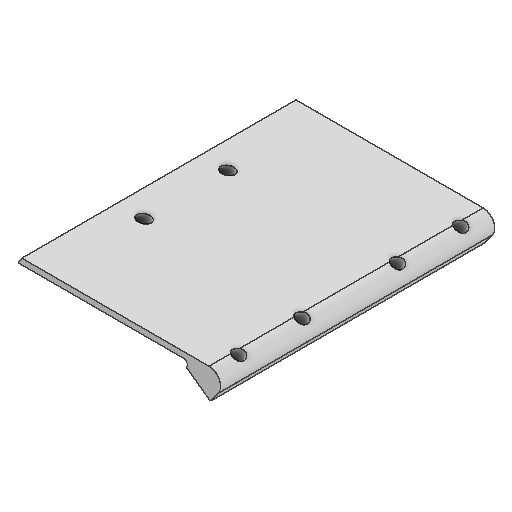
# Autodesk Inventor part: rearSkidPlate
Saved by Autodesk Inventor 2025 (Build 290162000, 162)
## iProperties
Created: 2025-01-06
Part Number: rearSkidPlate
Material: Generic
Document SubType Name: Modeling
Designer: derm
Density: 1 g/cm^3
Appearance: Default
Author: derm
Autodesk Inventor part; units mm, degrees
ref_plane "YZ Plane" through (0, 0, 0) normal (1, 0, 0) x (0, 1, 0)
sketch "Sketch1" plane through (0, 0, 0) normal (0, 1, 0) x (-1, 0, 0)
  line L0 (-60, 117) -> (60, 117)
  line L1 (60, 117) -> (60, -117)
  line L2 (60, -117) -> (-60, -117)
  line L3 (-60, -117) -> (-60, 117)
  line L4 (-60, 117) -> (60, -117) construction
  line L5 (60, 117) -> (-60, -117) construction
  point P0 (0, 0)
  dimension "d0" = 234
  dimension "d1" = 120
  constraints: 12 end point, 2 midpoint, 2 parallel, 1 horizontal, 1 perpendicular
  measures "d0" distance of L2.end L0.start
  measures "d1" distance of L1.end L2.end
extrude "Extrusion1" add sketch "Sketch1" along normal blind 5
sketch "Sketch2" plane through (60, 0, -117) normal (0, 0, -1) x (-1, 0, 0)
  line L0 (220.5261, -138.6359) -> (120, 0) projected
  line L1 (0, 0) -> (120, 0) projected
  line L2 (120, 0) -> (120, 5) projected
  line L3 (0, 5) -> (120, 5) projected
  line L4 (0, 0) -> (0, 5) projected
  line L5 (120, 0) -> (116.3745, 5)
  point P0 (60, 0)
  constraints: 2 end point, 1 point on line
extrude "Extrusion2" cut sketch "Sketch2" against normal through all contours L5 L3 L2
sketch "Sketch3" plane through (60, 0, -117) normal (0, 0, -1) x (-1, 0, 0)
  line L0 (120, 0) -> (116.3745, 5) projected
  line L1 (0, 5) -> (116.3745, 5) projected
  line L2 (0, 0) -> (0, 5) projected
  line L3 (0, 0) -> (120, 0) projected
  line L4 (-29.1464, -9.1279) -> (-26.3491, -7.0996) projected
  line L5 (-44.5674, -20.3098) -> (-40.8398, -25.4506) projected
  line L6 (0, 5) -> (-62.9198, 5)
  line L7 (0, 0) -> (-27.9195, 0)
  line L8 (-79.2318, 0) -> (-79.2318, 5)
  line L9 (-9.681, -25.1528) -> (-22.4191, -7.5856) projected
  line L10 (-22.4191, -7.5856) -> (-27.9195, 0)
  line L11 (-44.5674, -20.3098) -> (-62.9198, 5)
  line L12 (-24.0044, -5.3994) -> (-44.5674, -20.3098)
  line L13 (-8.3183, -25.4) -> (-8.3183, -2.8036) projected
  line L14 (-8.3183, 0) -> (-8.3183, -25.4)
  line L15 (-8.3183, -25.4) -> (-9.0939, -25.9624)
  line L16 (-9.0939, -25.9624) -> (-27.9195, 0)
  point P0 (60, 0)
  point P1 (-26.3491, -7.0996)
  constraints: 18 end point, 2 collinear, 2 horizontal, 2 perpendicular, 2 point on line
extrude "Extrusion3" add sketch "Sketch3" against normal up to surface (234 mm away) contours L7 L10 L12 L4 L11 L6 L2 | L14 L13 L15 L16 L9 L10 L7
fillet "Fillet1" radius 10 1 edges at (122.9198, 5, 0)
sketch "Sketch4" plane through (68.3183, 0, -117) normal (0, 0, -1) x (-1, 0, 0)
  arc A0 (-34.9981, 5) -> (-43.0938, -10.8703) centre (-34.9981, -5) ccw projected
  line L0 (-43.0938, -10.8703) -> (-36.2491, -20.3098) projected
  line L1 (-36.2491, -20.3098) -> (-15.6861, -5.3994) projected
  line L2 (-15.6861, -5.3994) -> (-0.7756, -25.9624) projected
  line L3 (-0.7756, -25.9624) -> (0, -25.4) projected
  line L4 (0, -25.4) -> (0, 0) projected
  line L5 (0, 0) -> (128.3183, 0) projected
  line L6 (128.3183, 0) -> (124.6928, 5) projected
  line L7 (124.6928, 5) -> (-34.9981, 5) projected
  line L8 (0, 0) -> (128.3183, 0) projected
  line L9 (0, 0) -> (-19.6012, 0)
  line L10 (-15.6861, -5.3994) -> (-19.6012, 0)
  point P0 (68.3183, 0)
  constraints: 4 end point, 1 horizontal
extrude "Extrusion4" cut sketch "Sketch4" against normal blind 44.45 contours L10 L9 L4 L3 L2
fillet "Fillet2" radius 3 1 edges at (87.9195, 0, -94.775)
mirror "Mirror1" about plane through (0, 0, 0) normal (0, 0, 1) of "Fillet2", "Extrusion4"
sketch "Sketch5" plane through (0, 0, 0) normal (0, 0, 1) x (1, 0, 0)
  line L0 (84.0044, -5.3994) -> (84.4672, -4.7611) projected
  arc A0 (84.4672, -4.7611) -> (82.0385, 0) centre (82.0385, -3) ccw projected
  line L1 (82.0385, 0) -> (-60, 0) projected
  line L2 (-60, 0) -> (-56.3745, 5) projected
  line L3 (-56.3745, 5) -> (103.3164, 5) projected
  arc A1 (111.4121, -10.8703) -> (103.3164, 5) centre (103.3164, -5) ccw projected
  line L4 (111.4121, -10.8703) -> (104.5674, -20.3098) projected
  line L5 (104.5674, -20.3098) -> (84.0044, -5.3994) projected
  line L6 (-59.5814, -11.3472) -> (-46.3045, -20.9744) projected
  line L7 (-52.9392, -0.4835) -> (-155.6686, -142.158) projected
  line L8 (-48.6719, -37.8674) -> (-54.5421, -45.963) projected
  line L9 (-54.5421, -45.963) -> (-39.8279, -25.6706)
  line L10 (-39.8279, -25.6706) -> (-60.391, -10.7602)
  line L11 (-60.391, -10.7602) -> (-52.5886, 0)
  line L12 (82.0385, 0) -> (-60, 0) projected
  line L13 (-39.8279, -25.6706) -> (-21.2139, 0)
  line L14 (-60, 0) -> (82.0385, 0) projected
  line L15 (-52.5886, 0) -> (-21.2139, 0)
  point P0 (0, 0)
  constraints: 10 end point, 3 point on line, 1 collinear, 1 perpendicular
extrude "Extrusion5" add sketch "Sketch5" along normal mid plane 101.6 contours L13 L10 L6 L7 L11 L1
sketch "Sketch6" plane through (-39.8279, -25.6706, -50.8) normal (-0.5870252, -0.8095687, 0) x (0.8095687, -0.5870252, 0)
  line L0 (0, 0) -> (0, 101.6) projected
  line L1 (-25.4, 101.6) -> (0, 101.6) projected
  line L2 (-25.4, 0) -> (-25.4, 101.6) projected
  line L3 (0, 0) -> (-25.4, 0) projected
  line L4 (88.351, 167.8) -> (113.751, 167.8) projected
  line L5 (88.351, 123.35) -> (88.351, 167.8) projected
  line L6 (88.351, -21.75) -> (88.351, 123.35) projected
  line L7 (88.351, -66.2) -> (88.351, -21.75) projected
  line L8 (113.751, -66.2) -> (88.351, -66.2) projected
  line L9 (113.751, -66.2) -> (113.751, 167.8) projected
  line L10 (113.751, 50.8) -> (-31.4, 50.8) construction
  line L11 (-31.4, -66.2) -> (-31.4, 167.8) projected
  circle A0 centre (-12.7, 86.5239) radius 2.75
  circle A1 centre (101.051, 145.575) radius 2.75
  circle A2 centre (101.051, 91.4911) radius 2.75
  circle A3 centre (-12.7, 15.0761) radius 2.75
  circle A4 centre (101.051, -43.975) radius 2.75
  circle A5 centre (101.051, 10.1089) radius 2.75
  point P0 (17.1741, 50.8)
  dimension "d14" = 5.5
  constraints: 6 centre point, 3 symmetric about line, 2 end point, 2 equal radius, 2 midpoint, 3 other
  measures "d14" diameter of A1
extrude "Extrusion6" cut sketch "Sketch6" against normal through all contours A0 | A1 | A2 | A3 | A4 | A5
ref_plane "Work Plane1" through (-36.8928, -21.6228, -50.8) normal (-0.5870252, -0.8095687, 0) x (0.8095687, -0.5870252, 0)
sketch "Sketch7" plane through (-36.8928, -21.6228, -50.8) normal (-0.5870252, -0.8095687, 0) x (0.8095687, -0.5870252, 0)
  circle A0 centre (-12.7, 15.0761) radius 2.75 projected
  circle A1 centre (-12.7, 86.5239) radius 2.75 projected
  line L0 (0, 0) -> (0, 101.6) projected
  line L1 (-25.4, 101.6) -> (0, 101.6) projected
  line L2 (-25.4, 0) -> (-25.4, 101.6) projected
  line L3 (0, 0) -> (-25.4, 0) projected
  circle A2 centre (-12.7, 86.5239) radius 5
  circle A3 centre (-12.7, 15.0761) radius 5
  point P0 (17.1741, 50.8)
  dimension "d18" = 10
  dimension "d19" = 10
  constraints: 2 centre point, 2 coincident
  measures "d18" diameter of A2
  measures "d19" diameter of A3
extrude "Extrusion7" cut sketch "Sketch7" against normal through all contours A2 | A3
ref_plane "Work Plane2" through (107.5026, -16.262, -117) normal (-0.5870252, -0.8095687, 0) x (0.8095687, -0.5870252, 0)
sketch "Sketch8" plane through (107.5026, -16.262, -117) normal (-0.5870252, -0.8095687, 0) x (0.8095687, -0.5870252, 0)
  circle A0 centre (-12.7, 76.3089) radius 2.75 projected
  circle A1 centre (-12.7, 157.6911) radius 2.75 projected
  circle A2 centre (-12.7, 22.225) radius 2.75 projected
  circle A3 centre (-12.7, 211.775) radius 2.75 projected
  line L0 (-25.4, 234) -> (0, 234) projected
  line L1 (-25.4, 189.55) -> (-25.4, 234) projected
  line L2 (-25.4, 44.45) -> (-25.4, 189.55) projected
  line L3 (-25.4, 0) -> (-25.4, 44.45) projected
  line L4 (0, 0) -> (-25.4, 0) projected
  line L5 (0, 0) -> (0, 234) projected
  circle A4 centre (-12.7, 211.775) radius 5
  circle A5 centre (-12.7, 157.6911) radius 5
  circle A6 centre (-12.7, 76.3089) radius 5
  circle A7 centre (-12.7, 22.225) radius 5
  point P0 (-96.5769, 117)
  dimension "d23" = 10
  constraints: 4 centre point, 4 coincident, 3 equal radius
  measures "d23" diameter of A4
extrude "Extrusion8" cut sketch "Sketch8" against normal through all contours A0 | A4 | A5 | A6 | A7
body "Solid1"
